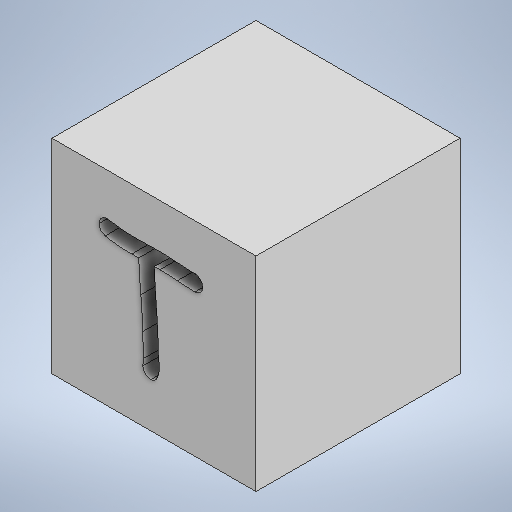
# Autodesk Inventor part: Thymine1
Saved by Autodesk Inventor 2025 (Build 290162000, 162)
## iProperties
Created: 2024-08-12
Part Number: Thymine1
Material: Generic
Document SubType Name: Modeling
Designer: kellst1
Density: 1 g/cm^3
Appearance: Default
Author: kellst1
Autodesk Inventor part; units mm, degrees
ref_plane "YZ Plane" through (0, 0, 0) normal (1, 0, 0) x (0, 1, 0)
ref_plane "XZ Plane" through (0, 0, 0) normal (0, 1, 0) x (-1, 0, 0)
ref_plane "XY Plane" through (0, 0, 0) normal (0, 0, 1) x (1, 0, 0)
sketch "Sketch1" plane through (0, 0, 0) normal (1, 0, 0) x (0, 1, 0)
  line L0 (0, 0) -> (10, 0)
  line L1 (10, 0) -> (10, -10)
  line L2 (10, -10) -> (0, -10)
  line L3 (0, -10) -> (0, 0)
  dimension "d0" = 10
  dimension "d1" = 10
  constraints: 8 end point, 2 parallel, 1 horizontal, 1 perpendicular
  measures "d0" distance of L1.end L2.end
  measures "d1" distance of L0.end L1.end
extrude "Extrusion1" add sketch "Sketch1" along normal blind 10
sketch "Sketch3" plane through (0, 0, 0) normal (-1, 0, 0) x (0, 0, 1)
  circle A0 centre (-5, 5) radius 1.5
  point P0 (0, 0)
  constraints: 1 centre point
extrude "Extrusion3" cut sketch "Sketch3" against normal blind 5
sketch "Sketch4" plane through (0, 0, 0) normal (0, 0, 1) x (1, 0, 0)
  line L0 (1.8731, 7.9408) -> (4.4271, 7.9408) construction
  line L1 (4.4271, 7.9408) -> (4.4271, 4.8928) construction
  line L2 (4.4271, 4.8928) -> (1.8731, 4.8928) construction
  line L3 (1.8731, 4.8928) -> (1.8731, 7.9408) construction
  spline S0 degree 2 poles (7.0108, 6.9784) (6.7321, 6.9784) (6.1484, 7.0258) knots 0 0 0 1 1 1
  spline S1 degree 2 poles (6.1484, 7.0258) (5.5857, 7.0678) (5.2912, 7.0626) knots 0 0 0 1 1 1
  line L4 (5.2912, 7.0626) -> (5.023, 7.0626)
  spline S2 degree 2 poles (5.023, 7.0626) (5.0336, 6.542) (5.1229, 5.3693) knots 0 0 0 1 1 1
  spline S3 degree 2 poles (5.1229, 5.3693) (5.2071, 4.2808) (5.2071, 3.676) knots 0 0 0 1 1 1
  spline S4 degree 2 poles (5.2071, 3.676) (5.2071, 3.5445) (5.2597, 3.0082) (5.2597, 2.8714) knots 0 0 0 1 2 2 2
  spline S5 degree 2 poles (5.2597, 2.8714) (5.2597, 2.619) (5.1755, 2.4297) knots 0 0 0 1 1 1
  spline S6 degree 2 poles (5.1755, 2.4297) (5.0704, 2.1826) (4.8495, 2.1826) knots 0 0 0 1 1 1
  spline S7 degree 2 poles (4.8495, 2.1826) (4.697, 2.1826) (4.4551, 2.3929) (4.4551, 2.5612) knots 0 0 0 1 2 2 2
  spline S8 degree 2 poles (4.4551, 2.5612) (4.4551, 2.619) (4.4919, 2.8452) (4.4919, 2.8977) knots 0 0 0 1 2 2 2
  spline S9 degree 2 poles (4.4919, 2.8977) (4.4919, 3.087) (4.4446, 3.8233) (4.4446, 4.0126) knots 0 0 0 1 2 2 2
  spline S10 degree 2 poles (4.4446, 4.0126) (4.4446, 4.5542) (4.3552, 5.5323) knots 0 0 0 1 1 1
  spline S11 degree 2 poles (4.3552, 5.5323) (4.2658, 6.584) (4.2553, 7.0468) knots 0 0 0 1 1 1
  line L5 (4.2553, 7.0468) -> (3.9135, 7.0415)
  spline S12 degree 2 poles (3.9135, 7.0415) (3.0879, 7.0415) (2.6146, 7.1625) knots 0 0 0 1 1 1
  spline S13 degree 2 poles (2.6146, 7.1625) (2.3096, 7.2414) (2.3096, 7.5358) knots 0 0 0 1 1 1
  spline S14 degree 2 poles (2.3096, 7.5358) (2.3096, 7.6936) (2.4095, 7.8093) knots 0 0 0 1 1 1
  spline S15 degree 2 poles (2.4095, 7.8093) (2.5199, 7.9408) (2.6987, 7.9302) knots 0 0 0 1 1 1
  spline S16 degree 2 poles (2.6987, 7.9302) (2.8302, 7.925) (3.3035, 7.8619) knots 0 0 0 1 1 1
  spline S17 degree 2 poles (3.3035, 7.8619) (3.6768, 7.8146) (3.9135, 7.8146) knots 0 0 0 1 1 1
  spline S18 degree 2 poles (3.9135, 7.8146) (4.1396, 7.8146) (5.0598, 7.8356) (5.286, 7.8356) knots 0 0 0 1 2 2 2
  spline S19 degree 2 poles (5.286, 7.8356) (5.5752, 7.8356) (6.7163, 7.7514) (7.0108, 7.7514) knots 0 0 0 1 2 2 2
  spline S20 degree 2 poles (7.0108, 7.7514) (7.1686, 7.7514) (7.3894, 7.5306) (7.3894, 7.3623) knots 0 0 0 1 2 2 2
  spline S21 degree 2 poles (7.3894, 7.3623) (7.3894, 7.2045) (7.1686, 6.9784) (7.0108, 6.9784) knots 0 0 0 1 2 2 2
  point P0 (0, 0)
  constraints: 2 other
extrude "Extrusion4" cut sketch "Sketch4" against normal blind 2
body "Solid1"
